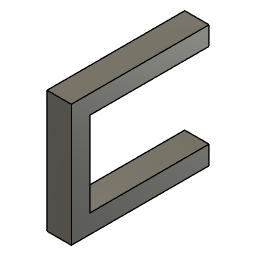
highway hackpad (Autodesk Fusion 360 design; units mm, degrees)
Autodesk Fusion 360 part; units mm, degrees
sketch "Sketch1" plane through (0, 0, 0) normal (1, 0, 0) x (0, 0, -1)
  line L0 (-25.4, 25.4) -> (25.4, 25.4)
  line L1 (25.4, 25.4) -> (25.4, -63.5)
  line L2 (25.4, -63.5) -> (-25.4, -63.5)
  line L3 (-25.4, -63.5) -> (-25.4, 25.4)
  constraint horizontal L0
  constraint vertical L1
  constraint horizontal L2
  constraint vertical L3
sketch "Sketch2" plane through (0, 0, 0) normal (1, 0, 0) x (0, 0, -1)
  line L0 (0, 0) -> (-89.049, 0)
  line L1 (-89.049, 0) -> (-89.049, -45.288)
  line L2 (-89.049, -45.288) -> (0, -45.288)
  line L3 (0, -45.288) -> (0, 0)
  line L4 (10, 10) -> (-99.049, 10)
  line L5 (-99.049, 10) -> (-99.049, -55.288)
  line L6 (-99.049, -55.288) -> (10, -55.288)
  line L7 (10, -55.288) -> (10, 10)
  line L8 (-25.4, -63.5) -> (-25.4, 25.4)
  dimension "d1" = 89.049
  dimension "d2" = 45.288
  dimension "d3" = 109.049
  dimension "d4" = 65.288
  dimension "d6" = 10
  dimension "d7" = 10
  dimension "d8" = 25.4
  constraint horizontal L0
  constraint vertical L1
  constraint horizontal L2
  constraint vertical L3
  constraint coincident L0.start L3.end
  constraint horizontal L4
  constraint vertical L5
  constraint horizontal L6
  constraint vertical L7
  measures "d1" distance of L0.start L0.end
  measures "d2" distance of L0.start L2.end
  measures "d3" distance of L4.start L4.end
  measures "d4" distance of L4.start L6.end
  measures "d6" distance of L2 L6
  measures "d7" distance of L3 L7
  measures "d8" distance of L3 L8
extrude "Extrude1" add sketch "Sketch2" along normal blind 13 contours L0 L2 L3 L4 L6 L7 L8 | L0 L1 L2 L4 L5 L6 L8
extrude "Extrude2" cut sketch "Sketch1" along normal blind 13
sketch "Sketch3" plane through (0, 0, 0) normal (1, 0, 0) x (0, 0, -1)
